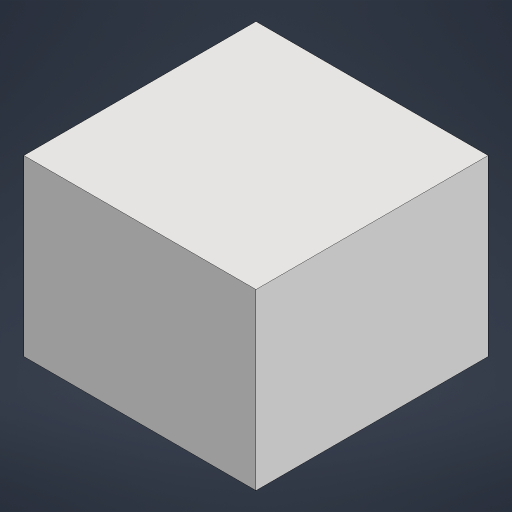
# Autodesk Inventor part: Setts
Saved by Autodesk Inventor 2023.1 (Build 271208000, 208)
## iProperties
RuleStatus: InUse
Created: 2022-11-16
Part Number: Setts
Material: Generic
Document SubType Name: Modeling
Designer: awelt
Mass: 786.579 g
Surface Area: 516.128 cm^2
Volume: 786.579 cm^3
Density: 1 g/cm^3
Appearance: Default
BeforeDocSave0: file://C:\Users\awelt\Documents\Inventor\iLogic_Rules\BoundingStore
DocClose0: file://C:\Users\awelt\Documents\Inventor\iLogic_Rules\BoundingStore
BoundingBL1: 3
BoundingBL2: 4
BoundingBL3: 4
BoundingCF: 0.028
Author: awelt
Autodesk Inventor part; units mm, degrees
ref_plane "YZ Plane" through (0, 0, 0) normal (1, 0, 0) x (0, 1, 0)
ref_plane "XZ Plane" through (0, 0, 0) normal (0, 1, 0) x (-1, 0, 0)
ref_plane "XY Plane" through (0, 0, 0) normal (0, 0, 1) x (1, 0, 0)
sketch "Sketch2" plane through (0, 0, 0) normal (0, 1, 0) x (-1, 0, 0)
  line L0 (0, 0) -> (-101.6, 0)
  line L1 (-101.6, 0) -> (-101.6, -101.6)
  line L2 (-101.6, -101.6) -> (0, -101.6)
  line L3 (0, -101.6) -> (0, 0)
  dimension "d3" = 101.6
  dimension "d4" = 101.6
  constraints: 8 end point, 2 parallel, 1 horizontal, 1 perpendicular
  measures "d3" distance of L2.end L1.end
  measures "d4" distance of L1.end L0.end
extrude "Extrusion1" add sketch "Sketch2" along normal blind 76.2
body "Solid1"
